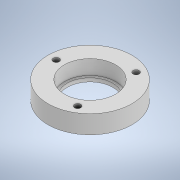
# Autodesk Inventor part: cazoleta
Saved by Autodesk Inventor 2021 (Build 250183000, 183)
## iProperties
Created: 2026-06-09
Part Number: cazoleta
Material: Generic
Document SubType Name: Modeling
Designer: nelso
Density: 1 g/cm^3
Appearance: Default
Author: nelso
Autodesk Inventor part; units mm, degrees
ref_plane "YZ Plane" through (0, 0, 0) normal (1, 0, 0) x (0, 1, 0)
ref_plane "XZ Plane" through (0, 0, 0) normal (0, 1, 0) x (-1, 0, 0)
ref_plane "XY Plane" through (0, 0, 0) normal (0, 0, 1) x (1, 0, 0)
sketch "Sketch1" plane through (0, 0, 0) normal (0, 1, 0) x (-1, 0, 0)
  circle A0 centre (0, 0) radius 14
  circle A1 centre (0, 0) radius 23
  line L0 (18.5, 0) -> (-9.25, -16.0215)
  line L1 (-9.25, -16.0215) -> (-9.25, 16.0215)
  line L2 (-9.25, 16.0215) -> (18.5, 0)
  circle A2 centre (0, 0) radius 12.5
  dimension "d0" = 28
  dimension "d1" = 46
  dimension "d2" = 18.5
  dimension "d3" = 25
  constraints: 7 coincident, 6 end point, 3 centre point, 7 other
  measures "d0" diameter of A0
  measures "d1" diameter of A1
  measures "d2" distance of point (0, 0) L0.start
  measures "d3" diameter of A2
extrude "Extrusion1" add sketch "Sketch1" along normal blind 10 contours A0 L2 L0 | A0 L1 L2 | L0 L1 A0 | A1
extrude "Extrusion2" add sketch "Sketch1" along normal blind 2 contours A0 L0 A2 L2 | L2 A2 A0 | A0 L0 A2 | L2 A2 L1 A0 | A0 L1 A2 L0 | L1 A2 A0
hole "Hole1" at (-18.5, 0, 0) at (9.25, 0, 16.0215) at (9.25, 0, -16.0215) direction (0, 1, 0) diameter 3.4 end through all clearance for "Countersunk Flat Head Screw ISO 2009/7046" size "M3" standard "ISO"
body "Solid1"
